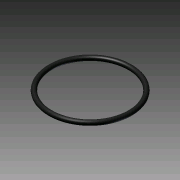
# Autodesk Inventor part: O-Ring 1764
Saved by Autodesk Inventor 2011 (Build 150239000, 239)
## iProperties
Created: 2010-01-18
Part Number: O-Ring 1764
Document SubType Name: Modeling
Designer: wbridges
Density: 1 g/cm^3
Author: wbridges
Autodesk Inventor part; units mm, degrees
ref_plane "YZ Plane" through (0, 0, 0) normal (1, 0, 0) x (0, 1, 0)
ref_plane "XZ Plane" through (0, 0, 0) normal (0, 1, 0) x (-1, 0, 0)
ref_plane "XY Plane" through (0, 0, 0) normal (0, 0, 1) x (1, 0, 0)
sketch "Sketch1" plane through (0, 0, 0) normal (0, 0, 1) x (1, 0, 0)
  circle A0 centre (16.8275, 0) radius 0.9525
  line L0 (0, 1.5875) -> (0, -5.4158)
  point P0 (0, 0)
  dimension "d2" = 1.905
  dimension "d3" = 16.8275
  constraints: 2 end point, 1 centre point, 1 horizontal alignment, 1 vertical
  measures "d2" diameter of A0
  measures "d3" distance of A0.centre point (0, 0)
revolve "Revolution1" add sketch "Sketch1" angle 360 about axis through (0, 1.5875, 0) along (0, -1, 0)
body "Solid1"
